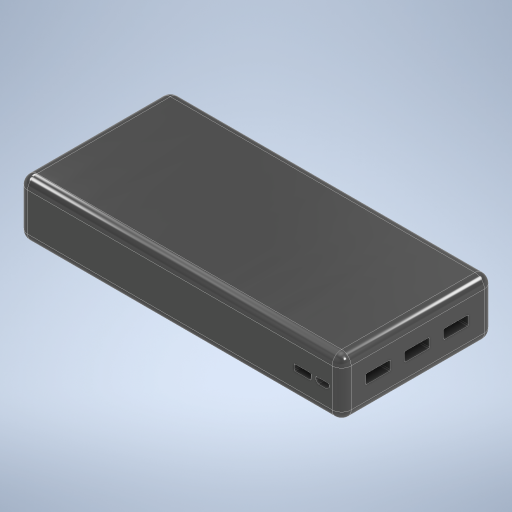
# Autodesk Inventor part: Large Battery
Saved by Autodesk Inventor 2024 (Build 280153000, 153)
## iProperties
Created: 2023-06-22
Part Number: Large Battery
Material: PET Plastic
Document SubType Name: Modeling
Designer: javie
Density: 1.541 g/cm^3
Appearance: Dark Gray
Author: javie
Autodesk Inventor part; units mm, degrees
ref_plane "YZ Plane" through (0, 0, 0) normal (1, 0, 0) x (0, 1, 0)
ref_plane "XZ Plane" through (0, 0, 0) normal (0, 1, 0) x (-1, 0, 0)
ref_plane "XY Plane" through (0, 0, 0) normal (0, 0, 1) x (1, 0, 0)
sketch "Sketch1" plane through (0, 0, 0) normal (0, 1, 0) x (-1, 0, 0)
  line L0 (170, 0) -> (0, 0)
  line L1 (0, 0) -> (0, -80)
  line L2 (0, -80) -> (170, -80)
  line L3 (170, -80) -> (170, 0)
  dimension "d1" = 170
  dimension "d2" = 80
  constraints: 8 end point, 2 parallel, 1 coincident, 1 horizontal, 1 perpendicular
  measures "d1" distance of L1.end L2.end
  measures "d2" distance of L0.end L1.end
extrude "Extrusion1" add sketch "Sketch1" along normal blind 30
fillet "Fillet1" radius 5 12 edges at (-85, 30, 0) (-85, 30, -80) (0, 30, -40) (-170, 30, -40) (-170, 0, -40) (-170, 15, 0) (-85, 0, 0) (-85, 0, -80) (0, 15, -80) (0, 0, -40) (-170, 15, -80) (0, 15, 0)
sketch "Sketch2" plane through (-165, 5, 0) normal (0, 0, 1) x (1, 0, 0)
  line L0 (148.44, 11.0782) -> (140.5, 11.0782)
  line L1 (140, 10.5782) -> (140, 8.3182)
  line L2 (140.5, 7.8182) -> (148.44, 7.8182)
  line L3 (148.94, 8.3182) -> (148.94, 10.5782)
  line L4 (0, 0) -> (0, 20) projected
  arc A0 (140.5, 11.0782) -> (140, 10.5782) centre (140.5, 10.5782) ccw
  arc A1 (140, 8.3182) -> (140.5, 7.8182) centre (140.5, 8.3182) ccw
  arc A2 (148.94, 10.5782) -> (148.44, 11.0782) centre (148.44, 10.5782) ccw
  arc A3 (148.44, 7.8182) -> (148.94, 8.3182) centre (148.44, 8.3182) ccw
  line L5 (151.9753, 11.0782) -> (157.8753, 11.0782)
  line L6 (158.3753, 10.5782) -> (158.3753, 9.3282)
  line L7 (156.8753, 8.0782) -> (152.7253, 8.0782)
  line L8 (151.4753, 9.3282) -> (151.4753, 10.5782)
  line L9 (151.4753, 8.0782) -> (151.4753, 8.0782)
  line L10 (151.4753, 8.0782) -> (151.4753, 8.0782) construction
  line L11 (157.1253, 8.0782) -> (156.8753, 8.0782)
  arc A4 (151.9753, 11.0782) -> (151.4753, 10.5782) centre (151.9753, 10.5782) ccw
  arc A5 (158.3753, 10.5782) -> (157.8753, 11.0782) centre (157.8753, 10.5782) ccw
  line L12 (151.4753, 9.3282) -> (152.7253, 8.0782)
  line L13 (151.4753, 9.3282) -> (153.243, 9.3282) construction
  line L14 (158.3753, 9.3282) -> (157.1253, 8.0782)
  point P0 (165, -5)
  point P1 (140, 7.8182)
  point P2 (140, 11.0782)
  point P3 (148.94, 7.8182)
  point P4 (158.3753, 11.0782)
  dimension "d6" = 8.94
  dimension "d7" = 3.26
  dimension "d8" = 140
  dimension "d9" = 0.5
  dimension "d12" = 45
  dimension "d13" = 0
  dimension "d14" = 1.25
  dimension "d15" = 0.5
  dimension "d16" = 6.9
  dimension "d17" = 45
  dimension "d18" = 3
  constraints: 28 end point, 12 point on circle, 12 tangent, 8 point on line, 6 centre point, 4 equal radius, 4 horizontal, 4 parallel, 2 equal length, 2 perpendicular
  measures "d6" distance of point (148.94, 7.818) point (140, 7.818)
  measures "d7" distance of point (140, 7.818) point (140, 11.078)
  measures "d8" distance between parallel lines of L4 L1
  measures "d9" radius of A0
  measures "d12" angle of L9 L10
  measures "d13" distance of L9.end L9.start
  measures "d14" vertical distance of L6.end L7.start
  measures "d15" radius of A4
  measures "d16" distance between parallel lines of L6 L8
  measures "d17" angle of L12 L13
  measures "d18" distance between parallel lines of L7 L5
extrude "Extrusion2" cut sketch "Sketch2" against normal blind 5
sketch "Sketch3" plane through (0, 5, -75) normal (1, 0, 0) x (0, 0, -1)
  line L0 (-61.8816, 12.5) -> (-49.8816, 12.5)
  line L1 (-49.3816, 12) -> (-49.3816, 8)
  line L2 (-49.8816, 7.5) -> (-61.8816, 7.5)
  line L3 (-62.3816, 8) -> (-62.3816, 12)
  line L4 (-41.3816, 12.5) -> (-29.3816, 12.5)
  line L5 (-28.8816, 12) -> (-28.8816, 8)
  line L6 (-29.3816, 7.5) -> (-41.3816, 7.5)
  line L7 (-41.8816, 8) -> (-41.8816, 12)
  line L8 (-20.8816, 12.5) -> (-8.8816, 12.5)
  line L9 (-8.3816, 12) -> (-8.3816, 8)
  line L10 (-8.8816, 7.5) -> (-20.8816, 7.5)
  line L11 (-21.3816, 8) -> (-21.3816, 12)
  line L12 (-75, 20) -> (-75, 0) projected
  line L13 (5, 0) -> (5, 20) projected
  line L14 (0, 25) -> (-70, 25) projected
  arc A0 (-61.8816, 12.5) -> (-62.3816, 12) centre (-61.8816, 12) ccw
  arc A1 (-49.3816, 12) -> (-49.8816, 12.5) centre (-49.8816, 12) ccw
  arc A2 (-62.3816, 8) -> (-61.8816, 7.5) centre (-61.8816, 8) ccw
  arc A3 (-49.8816, 7.5) -> (-49.3816, 8) centre (-49.8816, 8) ccw
  arc A4 (-41.3816, 12.5) -> (-41.8816, 12) centre (-41.3816, 12) ccw
  arc A5 (-28.8816, 12) -> (-29.3816, 12.5) centre (-29.3816, 12) ccw
  arc A6 (-41.8816, 8) -> (-41.3816, 7.5) centre (-41.3816, 8) ccw
  arc A7 (-29.3816, 7.5) -> (-28.8816, 8) centre (-29.3816, 8) ccw
  arc A8 (-20.8816, 12.5) -> (-21.3816, 12) centre (-20.8816, 12) ccw
  arc A9 (-8.3816, 12) -> (-8.8816, 12.5) centre (-8.8816, 12) ccw
  arc A10 (-21.3816, 8) -> (-20.8816, 7.5) centre (-20.8816, 8) ccw
  arc A11 (-8.8816, 7.5) -> (-8.3816, 8) centre (-8.8816, 8) ccw
  point P0 (-75, -5)
  point P1 (-49.3816, 7.5)
  point P2 (-49.3816, 12.5)
  point P3 (-62.3816, 7.5)
  point P4 (-28.8816, 7.5)
  point P5 (-28.8816, 12.5)
  point P6 (-41.8816, 7.5)
  point P7 (-8.3816, 7.5)
  point P8 (-8.3816, 12.5)
  point P9 (-21.3816, 7.5)
  point P10 (-49.3816, 10)
  point P11 (-21.3816, 10)
  point P12 (-28.8816, 10)
  point P13 (5, 10)
  point P14 (-62.3816, 10)
  dimension "d21" = 13
  dimension "d22" = 5
  dimension "d23" = 13
  dimension "d24" = 5
  dimension "d25" = 13
  dimension "d26" = 5
  dimension "d27" = 7.5
  dimension "d28" = 7.5
  dimension "d32" = 15
  dimension "d33" = 0.5
  constraints: 24 end point, 24 point on circle, 24 tangent, 18 point on line, 12 centre point, 11 equal radius, 6 parallel, 5 midpoint, 3 horizontal, 3 perpendicular, 2 collinear
  measures "d21" distance of point (-49.382, 7.5) point (-62.382, 7.5)
  measures "d22" distance of point (-49.382, 12.5) point (-49.382, 7.5)
  measures "d23" distance of point (-28.882, 7.5) point (-41.882, 7.5)
  measures "d24" distance of point (-28.882, 12.5) point (-28.882, 7.5)
  measures "d25" distance of point (-8.382, 7.5) point (-21.382, 7.5)
  measures "d26" distance of point (-8.382, 12.5) point (-8.382, 7.5)
  measures "d27" distance from line of L7 point (-49.382, 10)
  measures "d28" distance of point (-21.382, 10) point (-28.882, 10)
  measures "d32" distance from line of point (-62.382, 10) L14
  measures "d33" radius of A0
extrude "Extrusion3" cut sketch "Sketch3" against normal blind 5
sketch "Sketch4" plane through (-5, 5, -80) normal (0, 0, -1) x (-1, 0, 0)
  circle A0 centre (17.5, 10) radius 5
  line L0 (-5, 20) -> (-5, 0) projected
  line L1 (0, -5) -> (160, -5) projected
  circle A1 centre (17.5, 10) radius 4.5
  line L2 (17.5, 7.5) -> (17.5, 12.5) construction
  line L3 (19.5, 11.0782) -> (11.56, 11.0782) projected
  line L4 (17.75, 7.5) -> (17.75, 12.5)
  line L5 (17.25, 12.5) -> (17.25, 7.5)
  arc A2 (17.25, 7.5) -> (17.75, 7.5) centre (17.5, 7.5) ccw
  arc A3 (17.75, 12.5) -> (17.25, 12.5) centre (17.5, 12.5) ccw
  line L6 (17.5, 10) -> (22.5, 10) construction
  point P0 (-5, -5)
  dimension "d36" = 10
  dimension "d37" = 22.5
  dimension "d38" = 15
  dimension "d39" = 9
  dimension "d40" = 2.5
  dimension "d41" = 90
  dimension "d42" = 0.5
  constraints: 10 end point, 4 centre point, 4 point on circle, 4 tangent, 2 perpendicular, 1 coincident, 1 horizontal, 1 midpoint, 1 parallel
  measures "d36" diameter of A0
  measures "d37" distance from line of L0 A0.centre
  measures "d38" distance from line of A0.centre L1
  measures "d39" diameter of A1
  measures "d40" distance of L6.start L2.end
  measures "d41" angle of L6 L2
  measures "d42" diameter of A3
extrude "Extrusion4" cut sketch "Sketch4" against normal blind 0.5
body "Solid1"
